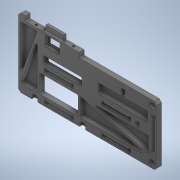
# Autodesk Inventor part: Cockpit_vertical_frame_01
Saved by Autodesk Inventor 2020 (Build 240168000, 168)
## iProperties
Created: 2021-08-10
Part Number: Cockpit_vertical_frame_01
Material: アセタール樹脂、黒
Document SubType Name: Modeling
Designer: Masato Kubotera
Density: 1.425 g/cm^3
Appearance: 滑らか - 黒
Mass: 38.105 g
Surface Area: 250.223 cm^2
Volume: 26.7404 cm^3
Description: POM T5
d0: 145.000 mm
d3: 81.000 mm
d4: 0.050 mm
d6: 2.100 mm
d7: 0.050 mm
d8: 0.050 mm
d9: 13.800 mm
d10: 9.200 mm
d11: 62.000 mm
d15: 2.500 mm
d16: 2.500 mm
d17: 5.000 mm
d21: 3.200 mm
d22: 6.000 mm
d23: 2.500 mm
d24: 5.000 mm
d25: 6.000 mm
d26: 3.200 mm
d27: 5.000 mm
d28: 2.500 mm
d29: 2.500 mm
d30: 5.000 mm
d31: 6.000 mm
d32: 3.200 mm
d33: 30.000 mm
d34: 2.500 mm
d35: 1.050 mm
d37: 0.050 mm
d38: 0.050 mm
d45: 30.000 mm
d46: 2.500 mm
d47: 1.050 mm
d48: 0.050 mm
d49: 0.050 mm
d55: 20.000 mm
d56: 10.000 mm
d57: 10.000 mm
d58: 2.500 mm
d59: 40.000 mm
d60: 30.000 mm
d71: 8.000 mm
d72: 12.000 mm
d73: 5.275 mm
d75: 40.000 mm
d76: 60.535 mm
d77: 30.000 mm
d78: 2.500 mm
d79: 1.050 mm
d80: 0.050 mm
d81: 0.050 mm
d82: 30.000 mm
d83: 2.500 mm
d84: 1.050 mm
d85: 0.050 mm
d86: 0.050 mm
d87: 1.050 mm
d88: 1.050 mm
d90: 18.833 mm
d91: 5.000 mm
d104: 28.250 mm
d105: 7.000 mm
d106: 2.100 mm
d107: 0.050 mm
d108: 0.050 mm
d109: 15.100 mm
d110: 10.600 mm
d121: 5.000 mm
d122: 0.00 deg
d123: 2.000 mm
d124: 0.00 deg
d125: 0.050 mm
d126: 0.050 mm
d127: 1.050 mm
d128: 2.500 mm
d129: 35.000 mm
d130: 2.500 mm
d133: 1.000 mm
Author: Masato Kubotera
Title: Cockpit_vertical_frame_01
Autodesk Inventor part; units mm, degrees
ref_plane "YZ Plane" through (0, 0, 0) normal (1, 0, 0) x (0, 1, 0)
ref_plane "XZ Plane" through (0, 0, 0) normal (0, 1, 0) x (-1, 0, 0)
ref_plane "XY Plane" through (0, 0, 0) normal (0, 0, 1) x (1, 0, 0)
sketch "スケッチ1" plane through (0, 0, 0) normal (0, 0, 1) x (1, 0, 0)
  line L0 (0, 0) -> (145, 0)
  line L1 (145, 0) -> (145, 62)
  line L2 (64, 67) -> (64, 62)
  line L3 (0, 67) -> (0, 0)
  line L4 (28.8, 64.65) -> (30.2849, 64.65) construction
  line L5 (42.7, 64.65) -> (42.7, 63.1651) construction
  line L6 (42.7, 55.35) -> (41.2151, 55.35) construction
  line L7 (28.8, 55.35) -> (28.8, 56.8349) construction
  line L8 (28.8, 64.65) -> (42.7, 55.35) construction
  line L9 (42.7, 64.65) -> (28.8, 55.35) construction
  line L10 (28.85, 64.6) -> (42.65, 64.6) construction
  line L11 (42.65, 64.6) -> (42.65, 55.4) construction
  line L12 (42.65, 55.4) -> (28.85, 55.4) construction
  line L13 (28.85, 55.4) -> (28.85, 64.6) construction
  line L14 (28.85, 64.6) -> (42.65, 55.4) construction
  line L15 (42.65, 64.6) -> (28.85, 55.4) construction
  arc A0 (30.2849, 64.65) -> (28.8, 63.1651) centre (29.5425, 63.9075) ccw
  line L16 (30.2849, 64.65) -> (28.8, 63.1651) construction
  line L17 (29.5425, 63.9075) -> (28.8, 64.65) construction
  line L18 (28.8, 60) -> (42.7, 60) construction
  line L19 (35.75, 64.65) -> (35.75, 55.35) construction
  arc A1 (42.7, 63.1651) -> (41.2151, 64.65) centre (41.9575, 63.9075) ccw
  arc A2 (28.8, 56.8349) -> (30.2849, 55.35) centre (29.5425, 56.0925) ccw
  arc A3 (41.2151, 55.35) -> (42.7, 56.8349) centre (41.9575, 56.0925) ccw
  line L20 (30.2849, 64.65) -> (41.2151, 64.65)
  line L21 (28.8, 63.1651) -> (28.8, 64.65) construction
  line L22 (41.2151, 64.65) -> (42.7, 64.65) construction
  line L23 (42.7, 63.1651) -> (42.7, 56.8349)
  line L24 (28.8, 56.8349) -> (28.8, 63.1651)
  line L25 (30.2849, 55.35) -> (28.8, 55.35) construction
  line L26 (41.2151, 55.35) -> (30.2849, 55.35)
  line L27 (42.7, 56.8349) -> (42.7, 55.35) construction
  line L28 (64, 62) -> (145, 62)
  line L29 (22.5, 27.9) -> (62.5, 27.9)
  line L30 (62.5, 27.9) -> (62.5, 8.6)
  line L31 (62.5, 8.6) -> (22.5, 8.6)
  line L32 (22.5, 8.6) -> (22.5, 27.9)
  line L33 (22.5, 27.9) -> (62.5, 8.6) construction
  line L34 (62.5, 27.9) -> (22.5, 8.6) construction
  line L35 (142.5, 62) -> (142.5, 0) construction
  line L36 (0, 36.5) -> (140, 36.5) construction
  line L37 (140, 31.5) -> (0, 31.5) construction
  line L38 (142.6289, 31) -> (142.5, 31) construction
  circle A4 centre (140, 5) radius 1.6
  circle A5 centre (140, 5) radius 3
  arc A6 (19.1583, 0) -> (15.8417, 0) centre (17.5, 2.5) ccw
  circle A7 centre (17.5, 2.5) radius 1.6
  line L39 (2.5, 31.5) -> (2.5, 0) construction
  line L40 (7.5, 0) -> (7.5, 31.5) construction
  line L41 (7.5, 5) -> (140, 5) construction
  arc A8 (69.1583, 0) -> (65.8417, 0) centre (67.5, 2.5) ccw
  circle A9 centre (67.5, 2.5) radius 1.6
  line L42 (27.5, 5) -> (57.5, 5) construction
  line L43 (57.5, 5) -> (57.5, 2.5) construction
  line L44 (57.5, 2.5) -> (27.5, 2.5) construction
  line L45 (27.5, 2.5) -> (27.5, 5) construction
  line L46 (27.5, 5) -> (57.5, 2.5) construction
  line L47 (57.5, 5) -> (27.5, 2.5) construction
  line L48 (27.45, 5.05) -> (29.55, 5.05) construction
  line L49 (57.55, 5.05) -> (57.55, 2.45)
  line L50 (57.55, 2.45) -> (55.45, 2.45) construction
  line L51 (27.45, 2.45) -> (27.45, 5.05)
  line L52 (27.45, 5.05) -> (57.55, 2.45) construction
  line L53 (57.55, 5.05) -> (27.45, 2.45) construction
  line L54 (27.45, 3.75) -> (57.55, 3.75) construction
  line L55 (42.5, 5.05) -> (42.5, 2.45) construction
  arc A10 (29.55, 5.05) -> (27.45, 5.05) centre (28.5, 5.05) ccw
  arc A11 (27.45, 2.45) -> (29.55, 2.45) centre (28.5, 2.45) ccw
  arc A12 (57.55, 5.05) -> (55.45, 5.05) centre (56.5, 5.05) ccw
  arc A13 (55.45, 2.45) -> (57.55, 2.45) centre (56.5, 2.45) ccw
  line L56 (29.55, 5.05) -> (55.45, 5.05)
  line L57 (29.55, 2.45) -> (27.45, 2.45) construction
  line L58 (55.45, 5.05) -> (57.55, 5.05) construction
  line L59 (55.45, 2.45) -> (29.55, 2.45)
  line L60 (87.5, 5) -> (117.5, 5) construction
  line L61 (117.5, 5) -> (117.5, 2.5) construction
  line L62 (117.5, 2.5) -> (87.5, 2.5) construction
  line L63 (87.5, 2.5) -> (87.5, 5) construction
  line L64 (87.5, 5) -> (117.5, 2.5) construction
  line L65 (117.5, 5) -> (87.5, 2.5) construction
  line L66 (87.45, 5.05) -> (89.55, 5.05) construction
  line L67 (117.55, 5.05) -> (117.55, 2.45)
  line L68 (117.55, 2.45) -> (115.45, 2.45) construction
  line L69 (87.45, 2.45) -> (87.45, 5.05)
  line L70 (87.45, 5.05) -> (117.55, 2.45) construction
  line L71 (117.55, 5.05) -> (87.45, 2.45) construction
  line L72 (87.45, 3.75) -> (117.55, 3.75) construction
  line L73 (102.5, 5.05) -> (102.5, 2.45) construction
  arc A14 (89.55, 5.05) -> (87.45, 5.05) centre (88.5, 5.05) ccw
  arc A15 (87.45, 2.45) -> (89.55, 2.45) centre (88.5, 2.45) ccw
  arc A16 (117.55, 5.05) -> (115.45, 5.05) centre (116.5, 5.05) ccw
  arc A17 (115.45, 2.45) -> (117.55, 2.45) centre (116.5, 2.45) ccw
  line L74 (89.55, 5.05) -> (115.45, 5.05)
  line L75 (89.55, 2.45) -> (87.45, 2.45) construction
  line L76 (115.45, 5.05) -> (117.55, 5.05) construction
  line L77 (115.45, 2.45) -> (89.55, 2.45)
  line L78 (54.535, 45.775) -> (66.535, 45.775)
  line L79 (66.535, 45.775) -> (66.535, 37.775)
  line L80 (66.535, 37.775) -> (54.535, 37.775)
  line L81 (54.535, 37.775) -> (54.535, 45.775) construction
  line L82 (54.535, 45.775) -> (66.535, 37.775) construction
  line L83 (66.535, 45.775) -> (54.535, 37.775) construction
  line L84 (26.535, 37.775) -> (26.535, 45.775)
  line L85 (26.535, 45.775) -> (54.535, 45.775)
  line L86 (54.535, 37.775) -> (26.535, 37.775)
  line L87 (54.535, 41.775) -> (66.535, 41.775) construction
  line L88 (55.45, 34.05) -> (57.55, 34.05) construction
  arc A18 (57.55, 34.05) -> (55.45, 34.05) centre (56.5, 34.05) ccw
  line L89 (57.5, 34) -> (57.5, 31.5) construction
  line L90 (57.55, 34.05) -> (57.55, 31.45)
  arc A19 (55.45, 31.45) -> (57.55, 31.45) centre (56.5, 31.45) ccw
  line L91 (57.55, 31.45) -> (55.45, 31.45) construction
  line L92 (27.5, 34) -> (57.5, 34) construction
  line L93 (42.5, 34.05) -> (42.5, 31.45) construction
  line L94 (29.55, 34.05) -> (55.45, 34.05)
  line L95 (55.45, 31.45) -> (29.55, 31.45)
  line L96 (27.45, 32.75) -> (57.55, 32.75) construction
  line L97 (27.45, 34.05) -> (57.55, 31.45) construction
  line L98 (57.55, 34.05) -> (27.45, 31.45) construction
  line L99 (57.5, 31.5) -> (27.5, 31.5) construction
  line L100 (27.5, 34) -> (57.5, 31.5) construction
  line L101 (57.5, 34) -> (27.5, 31.5) construction
  arc A20 (27.45, 31.45) -> (29.55, 31.45) centre (28.5, 31.45) ccw
  line L102 (29.55, 31.45) -> (27.45, 31.45) construction
  line L103 (27.5, 31.5) -> (27.5, 34) construction
  line L104 (27.45, 31.45) -> (27.45, 34.05)
  line L105 (27.45, 34.05) -> (29.55, 34.05) construction
  arc A21 (29.55, 34.05) -> (27.45, 34.05) centre (28.5, 34.05) ccw
  line L106 (115.45, 34.05) -> (117.55, 34.05) construction
  arc A22 (117.55, 34.05) -> (115.45, 34.05) centre (116.5, 34.05) ccw
  line L107 (117.5, 34) -> (117.5, 31.5) construction
  line L108 (117.55, 34.05) -> (117.55, 31.45)
  arc A23 (115.45, 31.45) -> (117.55, 31.45) centre (116.5, 31.45) ccw
  line L109 (117.55, 31.45) -> (115.45, 31.45) construction
  line L110 (87.5, 34) -> (117.5, 34) construction
  line L111 (102.5, 34.05) -> (102.5, 31.45) construction
  line L112 (89.55, 34.05) -> (115.45, 34.05)
  line L113 (115.45, 31.45) -> (89.55, 31.45)
  line L114 (87.45, 32.75) -> (117.55, 32.75) construction
  line L115 (87.45, 34.05) -> (117.55, 31.45) construction
  line L116 (117.55, 34.05) -> (87.45, 31.45) construction
  line L117 (117.5, 31.5) -> (87.5, 31.5) construction
  line L118 (87.5, 34) -> (117.5, 31.5) construction
  line L119 (117.5, 34) -> (87.5, 31.5) construction
  arc A24 (87.45, 31.45) -> (89.55, 31.45) centre (88.5, 31.45) ccw
  line L120 (89.55, 31.45) -> (87.45, 31.45) construction
  line L121 (87.5, 31.5) -> (87.5, 34) construction
  line L122 (87.45, 31.45) -> (87.45, 34.05)
  line L123 (87.45, 34.05) -> (89.55, 34.05) construction
  arc A25 (89.55, 34.05) -> (87.45, 34.05) centre (88.5, 34.05) ccw
  line L124 (26.3333, 72) -> (45.1667, 72)
  line L125 (26.3333, 72) -> (26.3333, 67)
  arc A26 (24.2333, 67) -> (26.3333, 67) centre (25.2833, 67) ccw
  line L126 (45.1667, 72) -> (45.1667, 67)
  line L127 (47.2667, 67) -> (64, 67)
  arc A27 (45.1667, 67) -> (47.2667, 67) centre (46.2167, 67) ccw
  line L128 (28.15, 65.35) -> (29.6349, 65.35) construction
  line L129 (43.35, 65.35) -> (43.35, 63.8651) construction
  line L130 (43.35, 54.65) -> (41.8651, 54.65) construction
  line L131 (28.15, 54.65) -> (28.15, 56.1349) construction
  line L132 (28.15, 65.35) -> (43.35, 54.65) construction
  line L133 (43.35, 65.35) -> (28.15, 54.65) construction
  line L134 (28.2, 65.3) -> (43.3, 65.3) construction
  line L135 (43.3, 65.3) -> (43.3, 54.7) construction
  line L136 (43.3, 54.7) -> (28.2, 54.7) construction
  line L137 (28.2, 54.7) -> (28.2, 65.3) construction
  line L138 (28.2, 65.3) -> (43.3, 54.7) construction
  line L139 (43.3, 65.3) -> (28.2, 54.7) construction
  arc A28 (29.6349, 65.35) -> (28.15, 63.8651) centre (28.8925, 64.6075) ccw
  line L140 (29.6349, 65.35) -> (28.15, 63.8651) construction
  line L141 (28.8925, 64.6075) -> (28.15, 65.35) construction
  line L142 (28.15, 60) -> (43.35, 60) construction
  line L143 (35.75, 65.35) -> (35.75, 54.65) construction
  arc A29 (43.35, 63.8651) -> (41.8651, 65.35) centre (42.6075, 64.6075) ccw
  arc A30 (28.15, 56.1349) -> (29.6349, 54.65) centre (28.8925, 55.3925) ccw
  arc A31 (41.8651, 54.65) -> (43.35, 56.1349) centre (42.6075, 55.3925) ccw
  line L144 (29.6349, 65.35) -> (41.8651, 65.35)
  line L145 (28.15, 63.8651) -> (28.15, 65.35) construction
  line L146 (41.8651, 65.35) -> (43.35, 65.35) construction
  line L147 (43.35, 63.8651) -> (43.35, 56.1349)
  line L148 (28.15, 56.1349) -> (28.15, 63.8651)
  line L149 (29.6349, 54.65) -> (28.15, 54.65) construction
  line L150 (41.8651, 54.65) -> (29.6349, 54.65)
  line L151 (43.35, 56.1349) -> (43.35, 54.65) construction
  line L152 (139.95, 48.55) -> (142.55, 48.55)
  line L153 (142.55, 48.55) -> (142.55, 46.45)
  line L154 (142.55, 13.45) -> (139.95, 13.45)
  line L155 (139.95, 13.45) -> (139.95, 15.55) construction
  line L156 (139.95, 48.55) -> (142.55, 13.45) construction
  line L157 (142.55, 48.55) -> (139.95, 13.45) construction
  line L158 (140, 48.5) -> (142.5, 48.5) construction
  line L159 (142.5, 48.5) -> (142.5, 13.5) construction
  line L160 (142.5, 13.5) -> (140, 13.5) construction
  line L161 (140, 13.5) -> (140, 48.5) construction
  line L162 (140, 48.5) -> (142.5, 13.5) construction
  line L163 (142.5, 48.5) -> (140, 13.5) construction
  line L164 (139.95, 31) -> (142.55, 31) construction
  line L165 (141.25, 48.55) -> (141.25, 13.45) construction
  arc A32 (139.95, 48.55) -> (139.95, 46.45) centre (139.95, 47.5) ccw
  arc A33 (142.55, 46.45) -> (142.55, 48.55) centre (142.55, 47.5) ccw
  arc A34 (139.95, 15.55) -> (139.95, 13.45) centre (139.95, 14.5) ccw
  arc A35 (142.55, 13.45) -> (142.55, 15.55) centre (142.55, 14.5) ccw
  line L166 (139.95, 46.45) -> (139.95, 48.55) construction
  line L167 (142.55, 46.45) -> (142.55, 15.55)
  line L168 (139.95, 15.55) -> (139.95, 46.45)
  line L169 (142.55, 15.55) -> (142.55, 13.45) construction
  line L170 (2.5, 59.5) -> (2.5, 67) construction
  line L171 (65, 27.9) -> (65, 8.6)
  line L172 (74.5806, 27.9) -> (75.3, 27.9) construction
  line L173 (65, 8.6) -> (136.4, 8.6)
  line L174 (136.4, 11.1897) -> (136.4, 27.9)
  line L175 (136.4, 27.9) -> (74.5806, 27.9)
  line L176 (65, 27.9) -> (136.4, 8.6)
  line L177 (74.5806, 27.9) -> (136.4, 11.1897)
  line L178 (2.5, 64.5) -> (20, 64.5)
  line L179 (20, 64.5) -> (2.5, 15.9699)
  line L180 (2.5, 15.9699) -> (2.5, 64.5)
  line L181 (20, 57.1301) -> (2.5, 8.6)
  line L182 (2.5, 8.6) -> (20, 8.6)
  line L183 (20, 8.6) -> (20, 57.1301)
  circle A36 centre (125, 32.75) radius 2
  line L184 (117.55, 32.75) -> (145, 32.75) construction
  line L185 (26.3333, 67) -> (45.1667, 67)
  line L186 (35.75, 72) -> (35.75, 67) construction
  line L187 (0, 67) -> (0, 72)
  line L188 (0, 72) -> (7.45, 72)
  line L189 (7.45, 72) -> (7.45, 68.4849)
  line L190 (7.5, 67) -> (7.5, 72) construction
  line L191 (7.45, 67) -> (8.9349, 67) construction
  arc A37 (7.45, 68.4849) -> (8.9349, 67) centre (8.1925, 67.7425) ccw
  line L192 (7.45, 68.4849) -> (7.45, 67) construction
  line L193 (8.9349, 67) -> (24.2333, 67)
  line L194 (84, 49.5) -> (85.4849, 49.5) construction
  line L195 (135.5, 49.5) -> (135.5, 48.0151) construction
  line L196 (135.5, 40) -> (134.0151, 40) construction
  line L197 (84, 40) -> (84, 41.4849) construction
  line L198 (109.75, 48.75) -> (109.75, 40) construction
  line L199 (84, 44.75) -> (135.5, 44.75) construction
  arc A38 (85.4849, 49.5) -> (84, 48.0151) centre (84.7425, 48.7575) ccw
  arc A39 (135.5, 48.0151) -> (134.0151, 49.5) centre (134.7575, 48.7575) ccw
  arc A40 (84, 41.4849) -> (85.4849, 40) centre (84.7425, 40.7425) ccw
  arc A41 (134.0151, 40) -> (135.5, 41.4849) centre (134.7575, 40.7425) ccw
  line L200 (84, 48.0151) -> (84, 49.5) construction
  line L201 (84, 41.4849) -> (84, 48.0151)
  line L202 (85.4849, 40) -> (84, 40) construction
  line L203 (134.0151, 40) -> (85.4849, 40)
  line L204 (135.5, 41.4849) -> (135.5, 40) construction
  line L205 (135.5, 48.0151) -> (135.5, 41.4849)
  line L206 (134.0151, 49.5) -> (135.5, 49.5) construction
  line L207 (85.4849, 49.5) -> (107.7, 49.5)
  line L208 (107.75, 53) -> (111.75, 53)
  line L209 (111.75, 53) -> (111.75, 57)
  line L210 (111.75, 57) -> (107.75, 57)
  line L211 (107.75, 57) -> (107.75, 53)
  line L212 (107.75, 53) -> (111.75, 57) construction
  line L213 (111.75, 53) -> (107.75, 57) construction
  line L214 (108.7, 53) -> (108.7, 50.5)
  line L215 (110.8, 53) -> (110.8, 50.5)
  line L216 (108.7, 49.5) -> (110.8, 49.5) construction
  line L217 (111.8, 49.5) -> (134.0151, 49.5)
  arc A42 (107.7, 49.5) -> (108.7, 50.5) centre (107.7, 50.5) ccw
  arc A43 (110.8, 50.5) -> (111.8, 49.5) centre (111.8, 50.5) ccw
  circle A44 centre (140, 57) radius 1.6
  circle A45 centre (140, 57) radius 3
  point P0 (35.75, 60)
  point P1 (35.75, 60)
  point P2 (42.5, 18.25)
  point P3 (42.5, 3.75)
  point P4 (102.5, 3.75)
  point P5 (42.5, 18.25)
  point P6 (60.535, 41.775)
  point P7 (42.5, 32.75)
  point P8 (102.5, 32.75)
  point P9 (35.75, 60)
  point P10 (35.75, 60)
  point P11 (141.25, 31)
  point P12 (141.25, 31)
  point P13 (109.75, 55)
  point P14 (109.75, 55)
  dimension "d0" = 145
  dimension "d3" = 81
  dimension "d6" = 2.1
  dimension "d7" = 0.05
  dimension "d8" = 0.05
  dimension "d9" = 13.8
  dimension "d10" = 9.2
  dimension "d11" = 62
  dimension "d15" = 2.5
  dimension "d17" = 5
  dimension "d21" = 3.2
  dimension "d22" = 6
  dimension "d23" = 2.5
  dimension "d24" = 5
  dimension "d25" = 6
  dimension "d26" = 3.2
  dimension "d28" = 2.5
  dimension "d29" = 2.5
  dimension "d30" = 5
  dimension "d31" = 6
  dimension "d32" = 3.2
  dimension "d33" = 30
  dimension "d34" = 2.5
  dimension "d35" = 1.05
  dimension "d37" = 0.05
  dimension "d38" = 0.05
  dimension "d45" = 30
  dimension "d46" = 2.5
  dimension "d47" = 1.05
  dimension "d48" = 0.05
  dimension "d49" = 0.05
  dimension "d55" = 20
  dimension "d56" = 10
  dimension "d57" = 10
  dimension "d58" = 2.5
  dimension "d59" = 40
  dimension "d60" = 30
  dimension "d71" = 8
  dimension "d72" = 12
  dimension "d73" = 5.275
  dimension "d75" = 40
  dimension "d76" = 60.535
  dimension "d77" = 30
  dimension "d78" = 2.5
  dimension "d79" = 1.05
  dimension "d80" = 0.05
  dimension "d81" = 0.05
  dimension "d82" = 30
  dimension "d83" = 2.5
  dimension "d84" = 1.05
  dimension "d85" = 0.05
  dimension "d86" = 0.05
  dimension "d87" = 1.05
  dimension "d88" = 1.05
  dimension "d90" = 18.8333
  dimension "d91" = 5
  dimension "d104" = 28.25
  dimension "d105" = 7
  dimension "d106" = 2.1
  dimension "d107" = 0.05
  dimension "d108" = 0.05
  dimension "d109" = 15.1
  dimension "d110" = 10.6
  dimension "d125" = 0.05
  constraints: 434 end point, 108 parallel, 93 perpendicular, 82 midpoint, 82 point on circle, 61 symmetric about line, 46 centre point, 43 horizontal, 27 point on line, 14 collinear, 8 vertical, 7 coincident, 4 tangent, 36 other
  measures "d0" distance of L1.start L3.end
  measures "d3" distance of L1.end L2.end
  measures "d6" diameter of A0
  measures "d7" distance from line of L19.start L10
  measures "d8" distance from line of L18.start L13
  measures "d9" distance of L10.end L10.start
  measures "d10" distance of L10.start L12.end
  measures "d11" distance of L1.start L1.end
  measures "d15" distance of L1.start L35.end
  measures "d17" distance of L37.end L36.start
  measures "d21" diameter of A4
  measures "d22" diameter of A5
  measures "d23" horizontal distance of A4.centre L35.end
  measures "d24" vertical distance of L35.end A4.centre
  measures "d25" diameter of A6
  measures "d26" diameter of A7
  measures "d28" vertical distance of L40.start A6.centre
  measures "d29" distance of L39.end L3.end
  measures "d30" distance of L40.start L39.end
  measures "d31" diameter of A8
  measures "d32" diameter of A9
  measures "d33" distance of L43.end L44.end
  measures "d34" distance of L42.end L43.end
  measures "d35" radius of A10
  measures "d37" distance from line of L45 L54.start
  measures "d38" distance from line of L42 L55.start
  measures "d45" distance of L61.end L62.end
  measures "d46" distance of L60.end L61.end
  measures "d47" radius of A14
  measures "d48" distance from line of L63 L72.start
  measures "d49" distance from line of L60 L73.start
  measures "d55" distance from line of L45 L41.start
  measures "d56" distance from line of L45 A6.centre
  measures "d57" distance from line of A8.centre L43
  measures "d58" vertical distance of L40.start A8.centre
  measures "d59" distance of L29.end L29.start
  measures "d60" distance between parallel lines of L63 L43
  measures "d71" distance of L79.end L78.end
  measures "d72" distance of L78.end L78.start
  measures "d73" distance from line of L36 point (60.535, 41.775)
  measures "d75" distance of L78.end L84.end
  measures "d76" horizontal distance of L3.start point (60.535, 41.775)
  measures "d77" distance of L89.end L101.end
  measures "d78" distance of L89.start L89.end
  measures "d79" radius of A21
  measures "d80" distance from line of L103 L96.start
  measures "d81" distance from line of L92 L93.start
  measures "d82" distance of L107.end L119.end
  measures "d83" distance of L107.start L107.end
  measures "d84" radius of A25
  measures "d85" distance from line of L121 L114.start
  measures "d86" distance from line of L110 L111.start
  measures "d87" radius of A26
  measures "d88" radius of A27
  measures "d90" distance of L2.start L126.end
  measures "d91" distance of L125.end L124.start
  measures "d104" distance between parallel lines of L2 L19
  measures "d105" distance between parallel lines of L127 L18
  measures "d106" diameter of A28
  measures "d107" distance from line of L143.start L134
  measures "d108" distance from line of L142.start L137
  measures "d109" distance of L134.end L134.start
  measures "d110" distance of L134.start L139.end
  measures "d125" distance from line of L158 L165.start
extrude "押し出し1" add sketch "スケッチ1" along normal blind 5 contours L3 L187 L188 L189 A37 L193 A26 L185 A27 L127 L2 L28 L1 L0 A8 A6
extrude "押し出し2" add sketch "スケッチ1" along normal blind 2 contours A6 L0 | A8 L0 | A5 | L144 A29 L147 A31 L150 A30 L148 A28 | A45
chamfer "面取り1" distance 2.5 angle 45 4 edges at (145, 62, 2.5) (145, 0, 2.5) (0, 0, 2.5) (0, 72, 2.5)
fillet "フィレット1" radius 1 29 edges at (15.8417, 0, 3.5) (19.1583, 0, 3.5) (65.8417, 0, 3.5) (69.1583, 0, 3.5) (26.535, 45.775, 2.5) (26.535, 37.775, 2.5) (66.535, 45.775, 2.5) (66.535, 37.775, 2.5) (22.5, 27.9, 2.5) (22.5, 8.6, 2.5) (62.5, 8.6, 2.5) (62.5, 27.9, 2.5) (64, 62, 2.5) (65, 27.9, 2.5) (65, 8.6, 2.5) (136.4, 8.6, 2.5) (136.4, 11.1897, 2.5) (136.4, 27.9, 2.5) (74.5806, 27.9, 2.5) (2.5, 15.9699, 2.5) (2.5, 8.6, 2.5) (20, 8.6, 2.5) (20, 57.1301, 2.5) (20, 64.5, 2.5) (2.5, 64.5, 2.5) (107.75, 57, 2.5) (111.75, 57, 2.5) (111.75, 53, 2.5) (107.75, 53, 2.5)
extrude "押し出し3" add sketch "スケッチ1" along normal blind 0.5 contours L176 L173 L171 | L177 L175 L174 | L178 L179 L180 | L183 L182 L181
extrude "押し出し4" add sketch "スケッチ1" along normal blind 2.5 contours L125 L124 L126 L185
sketch "スケッチ3" plane through (8.9349, 67, 0) normal (0, 1, 0) x (1, 0, 0)
  line L0 (36.2317, -2.5) -> (17.3984, -2.5) projected
  line L1 (26.8151, -2.5) -> (26.8151, 0)
  line L2 (17.3984, -2.5) -> (17.3984, -5) projected
  line L3 (15.2984, 0) -> (0, 0) projected
  point P0 (-8.9349, 0)
  point P1 (7.3984, -2.5)
  point P2 (46.2317, -2.5)
  dimension "d197" = 10
  dimension "d198" = 2.5
  constraints: 2 end point, 1 midpoint, 1 symmetric about line, 1 vertical
  measures "d197" distance from line of L2 point (7.398, -2.5)
  measures "d198" distance from line of point (7.398, -2.5) L3
hole "穴2" at (16.3333, 67, 2.5) at (55.1667, 67, 2.5) direction (0, -1, 0) diameter 2.459 depth 4 tip angle 118 thread size "M3x0.5" class "6H" standard "ISO Metric profile"
extrude "押し出し5" add sketch "スケッチ1" along normal blind 1 contours L207 A42 L214 L208 L215 A43 L217 A39 L205 A41 L203 A40 L201 A38
fillet "フィレット2" radius 2 2 edges at (108.7, 53.0013, 2.5) (110.8, 53.0013, 2.5)
equation "\"d7\" = d8"
equation "\"d25\" = d31"
equation "\"d26\" = d32"
equation "\"d28\" = 0.5 * d27"
equation "\"d31\" = d22"
equation "\"d32\" = d21"
equation "\"d38\" = d37"
equation "\"d27\" = 5"
